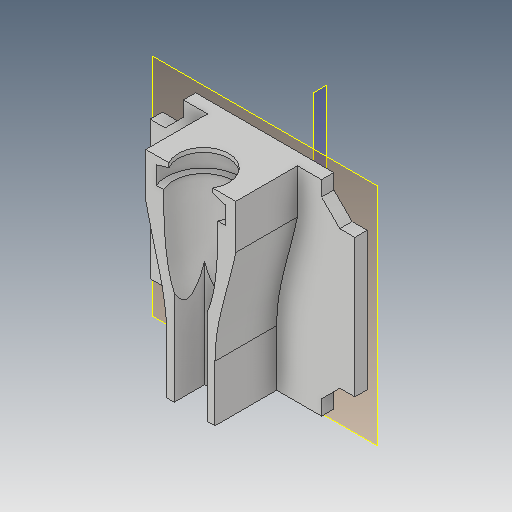
# Autodesk Inventor part: 20_Cube_Insert_Beamexpander
Saved by Autodesk Inventor 2019 (Build 230136000, 136)
## iProperties
Created: 2019-07-01
Part Number: 20_Cube_Insert_Beamexpander
Material: Generic
Document SubType Name: Modeling
Designer: diederichbenedict
Density: 1 g/cm^3
Appearance: Default
Author: diederichbenedict
Autodesk Inventor part; units mm, degrees
ref_plane "YZ Plane" through (0, 0, 0) normal (1, 0, 0) x (0, 1, 0)
ref_plane "XZ Plane" through (0, 0, 0) normal (0, 1, 0) x (-1, 0, 0)
ref_plane "XY Plane" through (0, 0, 0) normal (0, 0, 1) x (1, 0, 0)
ref_plane "Work Plane1" through (0, 0, 10) normal (0, 0, 1) x (1, 0, 0)
sketch "Sketch1" plane through (0, 0, 10) normal (0, 0, 1) x (1, 0, 0)
  line L0 (-4.0299, -0.3538) -> (-2.2322, 1.4439) construction
  arc A0 (-1.4439, 2.2322) -> (-2.2322, 1.4439) centre (-0.9299, 0.9299) ccw construction
  line L1 (-1.4439, 2.2322) -> (0.3538, 4.0299) construction
  line L2 (-37.8299, 42.2137) -> (-37.8299, 45.8299) construction
  line L3 (-37.8299, 45.8299) -> (-4.0299, 45.8299) construction
  line L4 (-4.0299, 45.8299) -> (-4.0299, 42.2137) construction
  line L5 (-4.0299, 4.0299) -> (0.3538, 4.0299) projected
  circle A1 centre (-20.9299, 20.9299) radius 17.5 projected
  line L6 (-20.9299, 58.9723) -> (17.1124, 20.9299) construction
  line L7 (17.1124, 20.9299) -> (-20.9299, -17.1124) construction
  line L8 (-20.9299, -17.1124) -> (-58.9723, 20.9299) construction
  line L9 (-58.9723, 20.9299) -> (-20.9299, 58.9723) construction
  line L10 (-20.9299, 58.9723) -> (-20.9299, -17.1124) construction
  line L11 (17.1124, 20.9299) -> (-58.9723, 20.9299) construction
  line L12 (-20.9299, 58.9723) -> (32.8701, 58.9723) construction
  line L13 (-43.4299, 43.4299) -> (1.5701, 43.4299) construction
  line L14 (1.5701, 43.4299) -> (1.5701, -1.5701) construction
  line L15 (1.5701, -1.5701) -> (-43.4299, -1.5701) construction
  line L16 (-43.4299, -1.5701) -> (-43.4299, 43.4299) construction
  line L17 (-43.4299, 43.4299) -> (1.5701, -1.5701) construction
  line L18 (1.5701, 43.4299) -> (-43.4299, -1.5701) construction
  line L19 (-43.4299, 5.3876) -> (-43.4299, 36.4723)
  line L20 (-43.4299, 36.4723) -> (-36.4723, 43.4299)
  line L21 (-36.4723, 43.4299) -> (-5.3876, 43.4299)
  line L22 (-5.3876, 43.4299) -> (1.5701, 36.4723)
  line L23 (1.5701, 36.4723) -> (1.5701, 5.3876)
  line L24 (1.5701, 5.3876) -> (-5.3876, -1.5701)
  line L25 (-5.3876, -1.5701) -> (-36.4723, -1.5701)
  line L26 (-36.4723, -1.5701) -> (-43.4299, 5.3876)
  line L27 (-4.0299, 42.2137) -> (-37.8299, 42.2137) projected
  line L28 (-4.0299, -0.3538) -> (-4.0299, 4.0299) projected
  circle A2 centre (-20.9299, 20.9299) radius 7.0417
  point P0 (-37.8299, 4.0299)
  dimension "d18" = 53.8
  dimension "d19" = 45
  dimension "d20" = 53.8
  dimension "d21" = 45
  dimension "d22" = 45
  constraints: 42 end point, 15 point on line, 5 midpoint, 4 parallel, 3 perpendicular, 2 horizontal, 1 centre point, 1 coincident, 1 equal length
  measures "d18" distance of L6.start L6.end
  measures "d19" angle of L6 L12
  measures "d20" distance of L6.end L7.end
  measures "d21" distance of L14.end L15.end
  measures "d22" distance of L13.end L14.end
extrude "Extrusion1" add sketch "Sketch1" along normal blind 3 contours L28 L24 L25 L26 L19 L20 L27 L22 L23 L5 | L5 L24 L28 | L27 L20 L21 L22 | A1
sketch "Sketch3" plane through (0, 0, 10) normal (0, 0, -1) x (-1, 0, 0)
  line L0 (37.8299, -0.4701) -> (37.8299, 4.0299) construction
  line L1 (4.0299, 4.0299) -> (4.0299, -0.4701) construction
  line L2 (37.8299, -0.4701) -> (37.8299, 1.1886) construction
  line L3 (4.0299, -3.9701) -> (4.0299, -0.3538) construction
  line L4 (45.8299, 4.0299) -> (42.2137, 4.0299) construction
  line L5 (-0.3538, 4.0299) -> (-3.9701, 4.0299) construction
  line L6 (-3.9701, 37.8299) -> (-0.3538, 37.8299) construction
  line L7 (4.0299, 42.2137) -> (4.0299, 45.8299) construction
  line L8 (37.8299, 45.8299) -> (37.8299, 42.2137) construction
  line L9 (42.2137, 37.8299) -> (45.8299, 37.8299) construction
  line L10 (37.8299, 37.7299) -> (45.8299, 37.7299)
  line L11 (45.8299, 37.7299) -> (45.8299, 4.1299)
  line L12 (45.8299, 4.1299) -> (37.8299, 4.1299)
  line L13 (37.8299, 4.1299) -> (37.8299, 37.7299)
  line L14 (37.7299, 4.0299) -> (4.1299, 4.0299)
  line L15 (4.1299, 4.0299) -> (4.1299, -3.9701)
  line L16 (4.1299, -3.9701) -> (37.7299, -3.9701)
  line L17 (37.7299, -3.9701) -> (37.7299, 4.0299)
  line L18 (4.0299, 4.1299) -> (-3.9701, 4.1299)
  line L19 (-3.9701, 4.1299) -> (-3.9701, 37.7299)
  line L20 (-3.9701, 37.7299) -> (4.0299, 37.7299)
  line L21 (4.0299, 37.7299) -> (4.0299, 4.1299)
  line L22 (4.1299, 37.8299) -> (37.7299, 37.8299)
  line L23 (37.7299, 37.8299) -> (37.7299, 45.8299)
  line L24 (37.7299, 45.8299) -> (4.1299, 45.8299)
  line L25 (4.1299, 45.8299) -> (4.1299, 37.8299)
  point P0 (0, 0)
  dimension "d23" = 0.1
  dimension "d24" = 0.1
  dimension "d25" = 0.1
  dimension "d26" = 0.1
  dimension "d27" = 0.1
  constraints: 32 end point, 8 parallel, 4 horizontal, 4 perpendicular, 3 point on line
  measures "d23" distance between parallel lines of L8 L23
  measures "d24" distance between parallel lines of L7 L25
  measures "d25" distance between parallel lines of L6 L20
  measures "d26" distance between parallel lines of L5 L18
  measures "d27" distance between parallel lines of L1 L15
extrude "Extrusion3" add sketch "Sketch3" against normal up to surface (3 mm away)
ref_plane "Work Plane4" through (-20.9299, 20.9299, 36.9) normal (-1, 0, 0) x (0, 1, 0)
sketch "Sketch11" plane through (-20.9299, 20.9299, 36.9) normal (-1, 0, 0) x (0, 1, 0)
  point P0 (-20.9299, 36.9)
sketch "Sketch12" plane through (0, 0, 13) normal (0, 0, 1) x (1, 0, 0)
  line L0 (-11.9799, 39.5299) -> (-11.9799, 43.8299) construction
  line L1 (-17.0799, -2.9701) -> (-17.0799, 2.0299) construction
  line L2 (-37.7299, 45.8299) -> (-4.1299, 45.8299) projected
  line L3 (-20.9299, 45.8299) -> (-20.9299, -3.9701)
  line L4 (-4.1299, -3.9701) -> (-37.7299, -3.9701) projected
  line L5 (-20.9299, -3.9701) -> (-15.0511, -3.9701)
  line L6 (-15.0511, -3.9701) -> (-15.0511, 9.6316)
  line L7 (-20.9299, 45.8299) -> (-9.9943, 45.8299)
  line L8 (-9.9943, 45.8299) -> (-9.9943, 35.0551)
  line L9 (-9.9943, 35.0551) -> (-12.2675, 24.6166) construction
  line L10 (-12.2675, 24.6166) -> (-15.0511, 18.1216) construction
  line L11 (-15.0511, 18.1216) -> (-15.0511, 9.6316) construction
  spline S0 degree 3 poles (-9.9943, 35.0551) (-12.2675, 24.6166) (-15.0511, 18.1216) (-15.0511, 9.6316) knots 1 1 1 1 2 2 2 2
  point P0 (0, 0)
  constraints: 12 end point, 3 vertical, 2 midpoint, 1 horizontal, 1 perpendicular, 1 point on line, 5 other
extrude "Extrusion10" add sketch "Sketch12" along normal blind 15
sketch "Sketch13" plane through (-20.9299, 13.8882, 13) normal (-1, 0, 0) x (0, 0, 1)
  line L0 (34.8, 31.9417) -> (-5, 31.9417) projected
  line L1 (36.8, -17.8583) -> (-5, -17.8583) construction
  line L2 (0, -17.8583) -> (15, -17.8583) projected
  line L3 (11.9179, -17.8583) -> (11.9179, 31.9417)
  line L4 (-5, 29.9417) -> (34.8, 29.9417) construction
  line L5 (16, -16.8583) -> (16, -11.8583) construction
  line L6 (9.0528, -16.8583) -> (9.0528, -11.8583) construction
  line L7 (9.709, -7.8145) -> (9.709, -17.8583)
  line L8 (9.709, -17.8583) -> (11.9179, -17.8583)
  arc A0 (5.7696, 30.9102) -> (2.95, 29.9417) centre (11.845, 8.6329) ccw
  line L9 (11.9179, 31.9417) -> (7.5, 31.9417)
  line L10 (0, 31.9417) -> (15, 31.9417) projected
  line L11 (9.709, -17.8583) -> (11.9179, -17.8583)
  line L12 (2.95, 29.9417) -> (2.95, 25.6417)
  line L13 (2.95, 25.6417) -> (4.6268, 25.6417)
  line L14 (7.5, 31.9417) -> (5.7696, 31.9417)
  line L15 (5.7696, 30.9102) -> (5.7696, 31.9417)
  line L16 (4.6268, 25.6417) -> (4.6268, 11.6155) construction
  line L17 (0, 21.1669) -> (15, 21.1669) projected
  line L18 (4.6268, 11.6155) -> (5.7696, 2.2174) construction
  line L19 (5.7696, 2.2174) -> (9.709, 3.7875) construction
  line L20 (9.709, 3.7875) -> (9.709, -7.8145) construction
  spline S0 degree 4 poles (4.6268, 25.6417) (4.6268, 11.6155) (5.7696, 2.2174) (9.709, 3.7875) (9.709, -7.8145) knots 1 1 1 1 1 2 2 2 2 2
  point P0 (-13, -13.8882)
  dimension "d69" = 4.4179
  constraints: 20 end point, 6 perpendicular, 4 point on line, 2 collinear, 2 point on circle, 2 vertical, 1 centre point, 1 midpoint, 6 other
  measures "d69" distance from line of L9.end L3
revolve "Revolution1" cut sketch "Sketch13" angle 360 about axis through (-20.9299, -3.9701, 24.9179) along (0, 1, 0)
sketch "Sketch14" plane through (-37.7299, -3.9701, 10) normal (0, -1, 0) x (1, 0, 0)
  circle A0 centre (16.8, 14.9) radius 2.8472 projected
  line L0 (12.95, 19) -> (20.65, 19) projected
  line L1 (12.95, 10.8) -> (12.95, 19) projected
  line L2 (20.65, 10.8) -> (12.95, 10.8) projected
  line L3 (20.65, 19) -> (20.65, 10.8) projected
  line L4 (20.85, 19.2) -> (12.75, 19.2)
  line L5 (12.75, 19.2) -> (12.75, 10.6)
  line L6 (12.75, 10.6) -> (20.85, 10.6)
  line L7 (20.85, 10.6) -> (20.85, 19.2)
  point P0 (37.7299, -10)
  dimension "d66" = 0.2
  constraints: 8 end point, 3 other
  measures "d66" distance between parallel lines of L0 L4
extrude "Extrusion11" cut sketch "Sketch14" against normal through all contours A0 | L0 L3 L2 L1 | L7 L6 L5 L4
mirror "Mirror1" about plane through (-20.9299, 45.8299, 13) normal (-1, 0, 0) of "Extrusion10", "Revolution1", "Extrusion11"
body "Solid1"
